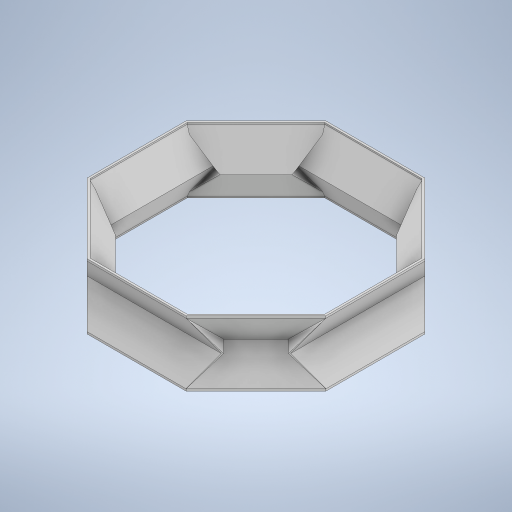
# Autodesk Inventor part: 팔각형 OV-PAM 층 한개
Saved by Autodesk Inventor 2024 (Build 280153000, 153)
## iProperties
Created: 2023-06-16
Part Number: 팔각형 OV-PAM 층 한개
Material: 일반
Document SubType Name: Modeling
Designer: jsw
Density: 1 g/cm^3
Appearance: 기본값
Author: jsw
Autodesk Inventor part; units mm, degrees
ref_plane "YZ Plane" through (0, 0, 0) normal (1, 0, 0) x (0, 1, 0)
ref_plane "XZ Plane" through (0, 0, 0) normal (0, 1, 0) x (-1, 0, 0)
ref_plane "XY Plane" through (0, 0, 0) normal (0, 0, 1) x (1, 0, 0)
sketch "스케치1" plane through (0, 0, 0) normal (0, 1, 0) x (-1, 0, 0)
  line L0 (-46.091883, 19.091883) -> (-19.091883, 46.091883)
  line L1 (-19.091883, 46.091883) -> (19.091883, 46.091883)
  line L2 (19.091883, 46.091883) -> (46.091883, 19.091883)
  line L3 (46.091883, 19.091883) -> (46.091883, -19.091883)
  line L4 (46.091883, -19.091883) -> (19.091883, -46.091883)
  line L5 (19.091883, -46.091883) -> (-19.091883, -46.091883)
  line L6 (-19.091883, -46.091883) -> (-46.091883, -19.091883)
  line L7 (-46.091883, -19.091883) -> (-46.091883, 19.091883)
  line L8 (-19.423254, 46.891883) -> (19.423254, 46.891883)
  line L9 (19.423254, 46.891883) -> (46.891883, 19.423254)
  line L10 (46.891883, 19.423254) -> (46.891883, -19.423254)
  line L11 (46.891883, -19.423254) -> (19.423254, -46.891883)
  line L12 (19.423254, -46.891883) -> (-19.423254, -46.891883)
  line L13 (-19.423254, -46.891883) -> (-46.891883, -19.423254)
  line L14 (-46.891883, -19.423254) -> (-46.891883, 19.423254)
  line L15 (-46.891883, 19.423254) -> (-19.423254, 46.891883)
  point P0 (0, 0)
  point P1 (0, 0)
  point P2 (0, 0)
  dimension "d0" = 38.18377
  dimension "d2" = 0.8
  constraints: 32 end point, 2 coincident, 2 horizontal, 34 other
  measures "d0" distance of L0.end L1.end
  measures "d2" distance between parallel lines of L10 L3
extrude "돌출2" add sketch "스케치1" along normal blind 12 contours L0 L1 L2 L3 L4 L5 L6 L7 | L8 L9 L10 L11 L12 L13 L14 L15
ref_plane "작업 평면2" through (46.891883, 0, 19.423254) normal (-0.8660254, -0.5, 0) x (0, 0, -1)
sketch "스케치3" plane through (46.891883, 0, 19.423254) normal (1, 0, 0) x (0, 0, -1)
  line L0 (0, 0) -> (0, 12)
  line L1 (0, 12) -> (38.846508, 12)
  line L2 (0, 0) -> (38.846508, 0)
  line L3 (38.846508, 0) -> (38.846508, 12)
  line L4 (38.846508, 12) -> (0, 12)
  line L5 (0, 12) -> (0, 0)
  line L6 (0, 12) -> (-7.304723, 12)
  line L7 (-27.468629, 12) -> (0, 12)
  line L8 (0, 0) -> (-7.304723, 12)
  line L9 (38.846508, 12) -> (46.151231, 12)
  line L10 (46.151231, 12) -> (38.846508, 0)
  point P0 (19.423254, 0)
  dimension "d17" = 121.33
  dimension "d18" = 121.33
  constraints: 16 end point, 2 parallel, 2 point on line, 1 horizontal, 1 perpendicular
  measures "d17" angle of L8 L2
  measures "d18" angle of L2 L10
extrude "돌출4" cut sketch "스케치3" against normal up to surface surface through (46.891883, 0, 19.423254) normal (-0.8660254, -0.5, 0)
sketch "스케치4" plane through (19.423254, 0, 46.891883) normal (0.7071068, 0, 0.7071068) x (0.7071068, 0, -0.7071068)
  line L0 (0, 0) -> (0, 12)
  line L1 (38.846508, 0) -> (38.846508, 12)
  line L2 (0, 0) -> (38.846508, 0)
  line L3 (38.846508, 0) -> (38.846508, 12)
  line L4 (38.846508, 12) -> (0, 12)
  line L5 (0, 12) -> (0, 0)
  line L6 (38.846508, 0) -> (29.048549, 12)
  line L7 (38.846508, 0) -> (28.423254, 12)
  line L8 (38.846508, 0) -> (0, 0)
  line L9 (0, 0) -> (10.423254, 12)
  line L10 (38.846508, 12) -> (0, 12)
  point P0 (19.423254, 0)
  point P1 (10.423254, 12)
  point P2 (19.423254, 12)
  dimension "d40" = 18
  dimension "d41" = 9
  constraints: 12 end point, 2 parallel, 2 point on line, 1 horizontal, 1 midpoint, 1 perpendicular
  measures "d40" distance of L9.end L7.end
  measures "d41" distance of L7.end point (19.423, 12)
ref_plane "작업 평면3" through (19.423254, 0, 46.891883) normal (0.6123724, 0.5, 0.6123724) x (0.7071068, 0, -0.7071068)
extrude "돌출5" cut sketch "스케치4" against normal up to surface contours L9 L4 L7 L2 surface through (19.423254, 0, 46.891883) normal (0.6123724, 0.5, 0.6123724)
pattern_circular "원형 패턴1" count 4 over 360 about axis through (0, -10, 0) along (0, 1, 0) of "돌출4"
pattern_circular "원형 패턴2" count 4 over 360 about axis through (0, -10, 0) along (0, 1, 0) of "돌출5"
mirror "미러5" about plane through (0, 12, 0) normal (0, 1, 0) of "돌출2", "돌출5", "원형 패턴2", "돌출4", "원형 패턴1"
ref_plane "작업 평면5" through (-19.423254, 12, -46.891883) normal (0, 1, 0) x (1, 0, 0)
sketch "스케치9" plane through (-19.423254, 24, -46.891883) normal (0, 1, 0) x (1, 0, 0)
  line L0 (66.315137, -66.315137) -> (66.315137, -27.468629)
  line L1 (66.315137, -27.468629) -> (38.846508, 0)
  line L2 (38.846508, 0) -> (0, 0)
  line L3 (0, 0) -> (-27.468629, -27.468629)
  line L4 (-27.468629, -27.468629) -> (-27.468629, -66.315137)
  line L5 (-27.468629, -66.315137) -> (0, -93.783766)
  line L6 (0, -93.783766) -> (38.846508, -93.783766)
  line L7 (38.846508, -93.783766) -> (66.315137, -66.315137)
  point P0 (19.423254, -46.891883)
extrude "돌출8" add sketch "스케치9" along normal blind 0.8
mirror "미러7" about plane through (-19.423254, 12, -46.891883) normal (0, 1, 0) of "돌출8"
shell "쉘5" thickness 0.8 removed faces 2 at (2.681792, 24.8, -6.474418) at (2.681792, -0.8, -6.474418)
equation "\"d41\" = 0.5 * d40"
